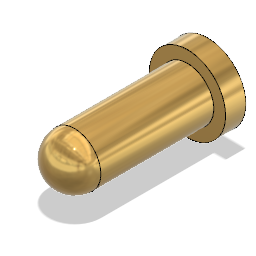
alum carriage v8 (Autodesk Fusion 360 archive; units mm, degrees)
design "brass pin"
Autodesk Fusion 360 part; units mm, degrees
sketch "Esquisse1" plane through (0, 0, 0) normal (0, 0, 1) x (1, 0, 0)
  circle A0 centre (0, 0) radius 1
  dimension "d1" = 2
  constraint coincident A0.centre origin
  measures "d1" diameter of A0
extrude "Extrusion1" add sketch "Esquisse1" along normal blind 4.3
sketch "Esquisse2" plane through (0, 0, 4.3) normal (0, 0, 1) x (1, 0, 0)
  circle A0 centre (0, 0) radius 1
  circle A1 centre (0, 0) radius 2.25
  dimension "d4" = 4.5
  constraint coincident A0.centre A1.centre
  measures "d4" diameter of A1
extrude "Extrusion2" add sketch "Esquisse2" along normal blind 1.2 contours A0 | A1
sketch "Esquisse3" plane through (0, 0, 5.5) normal (0, 0, 1) x (1, 0, 0)
  circle A0 centre (0, 0) radius 2.25
  circle A1 centre (0, 0) radius 1.55
  dimension "d7" = 3.1
  constraint coincident A0.centre A1.centre
  measures "d7" diameter of A1
extrude "Extrusion3" add sketch "Esquisse3" along normal blind 8.7 contours A1
extrude "Extrusion4" cut 1 faces at (-0.3296, 0.5031, 0) along direction (0, 0, 1) blind 4.3
extrude "Extrude5" cut 1 faces at (0.8338, -0.7144, 14.2) along direction (0, 0, -1) blind 0.5
fillet "Fillet2" radius 1.55 1 edges at (-1.4451, 0.5605, 13.7)
